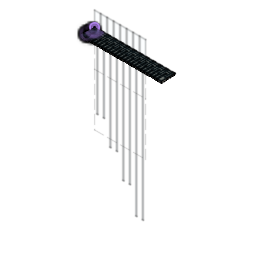
model (Autodesk Fusion 360 design; units mm, degrees)
Autodesk Fusion 360 part; units mm, degrees
sketch "kre" plane through (0, 0, 0) normal (0, 1, 0) x (1, 0, 0) in component "sketches"
  line L0 (20.5, 670) -> (29.5, 670)
  line L1 (29.5, 670) -> (29.5, 0)
  line L2 (29.5, 0) -> (20.5, 0)
  line L3 (20.5, 0) -> (20.5, 670)
  line L4 (0, 0) -> (50, 0)
  line L5 (50, 0) -> (50, -135)
  line L6 (50, -135) -> (0, -135)
  line L7 (0, -135) -> (0, 0)
  line L8 (109, 0) -> (109, -135)
  line L9 (109, -135) -> (59, -135)
  line L10 (59, -135) -> (59, 0)
  line L11 (59, 0) -> (109, 0)
  line L12 (88.5, 670) -> (88.5, 0)
  line L13 (88.5, 0) -> (79.5, 0)
  line L14 (79.5, 670) -> (88.5, 670)
  line L15 (79.5, 0) -> (79.5, 670)
  line L16 (168, 0) -> (168, -135)
  line L17 (168, -135) -> (118, -135)
  line L18 (118, -135) -> (118, 0)
  line L19 (118, 0) -> (168, 0)
  line L20 (147.5, 872) -> (147.5, 0)
  line L21 (147.5, 0) -> (138.5, 0)
  line L22 (138.5, 872) -> (147.5, 872)
  line L23 (138.5, 0) -> (138.5, 872)
  line L24 (227, 0) -> (227, -135)
  line L25 (227, -135) -> (177, -135)
  line L26 (177, -135) -> (177, 0)
  line L27 (177, 0) -> (227, 0)
  line L28 (206.5, 872) -> (206.5, 0)
  line L29 (206.5, 0) -> (197.5, 0)
  line L30 (197.5, 872) -> (206.5, 872)
  line L31 (197.5, 0) -> (197.5, 872)
  line L32 (286, 0) -> (286, -135)
  line L33 (286, -135) -> (236, -135)
  line L34 (236, -135) -> (236, 0)
  line L35 (236, 0) -> (286, 0)
  line L36 (265.5, 1074) -> (265.5, 0)
  line L37 (265.5, 0) -> (256.5, 0)
  line L38 (256.5, 1074) -> (265.5, 1074)
  line L39 (256.5, 0) -> (256.5, 1074)
  line L40 (345, 0) -> (345, -135)
  line L41 (345, -135) -> (295, -135)
  line L42 (295, -135) -> (295, 0)
  line L43 (295, 0) -> (345, 0)
  line L44 (324.5, 1074) -> (324.5, 0)
  line L45 (324.5, 0) -> (315.5, 0)
  line L46 (315.5, 1074) -> (324.5, 1074)
  line L47 (315.5, 0) -> (315.5, 1074)
  line L48 (404, 0) -> (404, -135)
  line L49 (404, -135) -> (354, -135)
  line L50 (354, -135) -> (354, 0)
  line L51 (354, 0) -> (404, 0)
  line L52 (383.5, 1295) -> (383.5, 0)
  line L53 (383.5, 0) -> (374.5, 0)
  line L54 (374.5, 1295) -> (383.5, 1295)
  line L55 (374.5, 0) -> (374.5, 1295)
  line L56 (463, 0) -> (463, -135)
  line L57 (463, -135) -> (413, -135)
  line L58 (413, -135) -> (413, 0)
  line L59 (413, 0) -> (463, 0)
  line L60 (442.5, 1295) -> (442.5, 0)
  line L61 (442.5, 0) -> (433.5, 0)
  line L62 (433.5, 1295) -> (442.5, 1295)
  line L63 (433.5, 0) -> (433.5, 1295)
  line L64 (50, 0) -> (59, 0) construction
  line L65 (109, 0) -> (118, 0) construction
  line L66 (168, 0) -> (177, 0) construction
  line L67 (227, 0) -> (236, 0) construction
  line L68 (286, 0) -> (295, 0) construction
  line L69 (345, 0) -> (354, 0) construction
  line L70 (404, 0) -> (413, 0) construction
  line L71 (0, 0) -> (463, 0) construction
  line L72 (463, 0) -> (463, 130) construction
  line L73 (463, 130) -> (0, 130) construction
  line L74 (0, 130) -> (0, 0) construction
  line L75 (0, 130) -> (0, 330) construction
  line L76 (0, 330) -> (463, 330) construction
  line L77 (463, 330) -> (463, 130) construction
  line L78 (0, 330) -> (0, 807) construction
  line L79 (0, 807) -> (463, 807) construction
  line L80 (463, 807) -> (463, 330) construction
  dimension "d1" = 135
  dimension "d2" = 50
  dimension "d3" = 805
  dimension "d4" = 9
  dimension "d5" = 135
  dimension "d6" = 50
  dimension "d7" = 805
  dimension "d8" = 9
  dimension "d9" = 135
  dimension "d10" = 50
  dimension "d11" = 1007
  dimension "d12" = 9
  dimension "d13" = 135
  dimension "d14" = 50
  dimension "d15" = 1007
  dimension "d16" = 9
  dimension "d17" = 135
  dimension "d18" = 50
  dimension "d19" = 1209
  dimension "d20" = 9
  dimension "d21" = 135
  dimension "d22" = 50
  dimension "d23" = 1209
  dimension "d24" = 9
  dimension "d25" = 135
  dimension "d26" = 50
  dimension "d27" = 1430
  dimension "d28" = 9
  dimension "d29" = 135
  dimension "d30" = 50
  dimension "d31" = 1430
  dimension "d32" = 9
  dimension "d34" = 50
  dimension "d35" = 130
  dimension "d56" = 200
  dimension "d57" = 677
  constraint horizontal L0
  constraint vertical L1
  constraint horizontal L2
  constraint vertical L3
  constraint horizontal L4
  constraint vertical L5
  constraint horizontal L6
  constraint vertical L7
  constraint midpoint L2 L4
  constraint horizontal L14
  constraint vertical L12
  constraint horizontal L13
  constraint vertical L15
  constraint horizontal L11
  constraint vertical L8
  constraint horizontal L9
  constraint vertical L10
  constraint midpoint L11 L13
  constraint horizontal L22
  constraint vertical L20
  constraint horizontal L21
  constraint vertical L23
  constraint horizontal L19
  constraint vertical L16
  constraint horizontal L17
  constraint vertical L18
  constraint midpoint L19 L21
  constraint horizontal L30
  constraint vertical L28
  constraint horizontal L29
  constraint vertical L31
  constraint horizontal L27
  constraint vertical L24
  constraint horizontal L25
  constraint vertical L26
  constraint midpoint L27 L29
  constraint horizontal L38
  constraint vertical L36
  constraint horizontal L37
  constraint vertical L39
  constraint horizontal L35
  constraint vertical L32
  constraint horizontal L33
  constraint vertical L34
  constraint midpoint L35 L37
  constraint horizontal L46
  constraint vertical L44
  constraint horizontal L45
  constraint vertical L47
  constraint horizontal L43
  constraint vertical L40
  constraint horizontal L41
  constraint vertical L42
  constraint midpoint L43 L45
  constraint horizontal L54
  constraint vertical L52
  constraint horizontal L53
  constraint vertical L55
  constraint horizontal L51
  constraint vertical L48
  constraint horizontal L49
  constraint vertical L50
  constraint midpoint L51 L53
  constraint horizontal L62
  constraint vertical L60
  constraint horizontal L61
  constraint vertical L63
  constraint horizontal L59
  constraint vertical L56
  constraint horizontal L57
  constraint vertical L58
  constraint midpoint L59 L61
  constraint collinear L6 L9
  constraint collinear L9 L17
  constraint collinear L17 L25
  constraint collinear L25 L33
  constraint collinear L33 L41
  constraint collinear L41 L49
  constraint collinear L49 L57
  constraint coincident L4.start L7.end
  constraint equal L64 L65
  constraint equal L65 L66
  constraint equal L66 L67
  constraint equal L67 L68
  constraint equal L68 L69
  constraint equal L69 L70
  constraint horizontal L71
  constraint vertical L72
  constraint horizontal L73
  constraint vertical L74
  constraint collinear L56 L72
  constraint vertical L77
  constraint vertical L75
  constraint horizontal L76
  constraint horizontal L79
  constraint vertical L80
  constraint vertical L78
  measures "d1" distance of L4.end L5.end
  measures "d2" distance of L5.end L6.end
  measures "d3" distance of L0 L6
  measures "d4" distance of L1 L3
  measures "d5" distance of L8.start L8.end
  measures "d6" distance of L9.end L8.end
  measures "d7" distance of L9 L14
  measures "d8" distance of L12 L15
  measures "d9" distance of L16.start L16.end
  measures "d10" distance of L17.end L16.end
  measures "d11" distance of L17 L22
  measures "d12" distance of L20 L23
  measures "d13" distance of L24.start L24.end
  measures "d14" distance of L25.end L24.end
  measures "d15" distance of L25 L30
  measures "d16" distance of L28 L31
  measures "d17" distance of L32.start L32.end
  measures "d18" distance of L33.end L32.end
  measures "d19" distance of L33 L38
  measures "d20" distance of L36 L39
  measures "d21" distance of L40.start L40.end
  measures "d22" distance of L41.end L40.end
  measures "d23" distance of L41 L46
  measures "d24" distance of L44 L47
  measures "d25" distance of L48.start L48.end
  measures "d26" distance of L49.end L48.end
  measures "d27" distance of L49 L54
  measures "d28" distance of L52 L55
  measures "d29" distance of L56.start L56.end
  measures "d30" distance of L57.end L56.end
  measures "d31" distance of L57 L62
  measures "d32" distance of L60 L63
  measures "d34" distance of L1 L15
  measures "d35" distance of L56.start L72.end
  measures "d56" distance of L73 L76
  measures "d57" distance of L73 L79
sketch "profile" plane through (0, 0, 0) normal (0, 0, 1) x (1, 0, 0) in component "rack"
  line L0 (0, 0) -> (726, 0)
  line L1 (726, 0) -> (726, -120)
  line L2 (726, -120) -> (0, -120)
  line L3 (0, -120) -> (0, 0)
  line L4 (33.5, -120) -> (43.5, -120)
  line L5 (43.5, -120) -> (43.5, -40)
  line L6 (43.5, -40) -> (33.5, -40)
  line L7 (33.5, -40) -> (33.5, -120)
  line L8 (92.5, -40) -> (92.5, -120)
  line L9 (92.5, -120) -> (102.5, -120)
  line L10 (102.5, -40) -> (92.5, -40)
  line L11 (102.5, -120) -> (102.5, -40)
  line L12 (151.5, -40) -> (151.5, -120)
  line L13 (151.5, -120) -> (161.5, -120)
  line L14 (161.5, -40) -> (151.5, -40)
  line L15 (161.5, -120) -> (161.5, -40)
  line L16 (210.5, -40) -> (210.5, -120)
  line L17 (210.5, -120) -> (220.5, -120)
  line L18 (220.5, -40) -> (210.5, -40)
  line L19 (220.5, -120) -> (220.5, -40)
  line L20 (269.5, -40) -> (269.5, -120)
  line L21 (269.5, -120) -> (279.5, -120)
  line L22 (279.5, -40) -> (269.5, -40)
  line L23 (279.5, -120) -> (279.5, -40)
  line L24 (328.5, -40) -> (328.5, -120)
  line L25 (328.5, -120) -> (338.5, -120)
  line L26 (338.5, -40) -> (328.5, -40)
  line L27 (338.5, -120) -> (338.5, -40)
  line L28 (387.5, -40) -> (387.5, -120)
  line L29 (387.5, -120) -> (397.5, -120)
  line L30 (397.5, -40) -> (387.5, -40)
  line L31 (397.5, -120) -> (397.5, -40)
  line L32 (446.5, -40) -> (446.5, -120)
  line L33 (446.5, -120) -> (456.5, -120)
  line L34 (456.5, -40) -> (446.5, -40)
  line L35 (456.5, -120) -> (456.5, -40)
  line L36 (505.5, -40) -> (505.5, -120)
  line L37 (505.5, -120) -> (515.5, -120)
  line L38 (515.5, -40) -> (505.5, -40)
  line L39 (515.5, -120) -> (515.5, -40)
  line L40 (564.5, -40) -> (564.5, -120)
  line L41 (564.5, -120) -> (574.5, -120)
  line L42 (574.5, -40) -> (564.5, -40)
  line L43 (574.5, -120) -> (574.5, -40)
  line L44 (623.5, -40) -> (623.5, -120)
  line L45 (623.5, -120) -> (633.5, -120)
  line L46 (633.5, -40) -> (623.5, -40)
  line L47 (633.5, -120) -> (633.5, -40)
  line L48 (682.5, -40) -> (682.5, -120)
  line L49 (682.5, -120) -> (692.5, -120)
  line L50 (692.5, -40) -> (682.5, -40)
  line L51 (692.5, -120) -> (692.5, -40)
  line L52 (63.75, -120) -> (72.25, -120)
  line L53 (72.25, -120) -> (72.25, -75)
  line L54 (72.25, -75) -> (63.75, -75)
  line L55 (63.75, -75) -> (63.75, -120)
  line L56 (63.75, -97.5) -> (43.5, -97.5) construction
  line L57 (72.25, -97.5) -> (92.5, -97.5) construction
  line L58 (122.75, -75) -> (122.75, -120)
  line L59 (122.75, -120) -> (131.25, -120)
  line L60 (131.25, -75) -> (122.75, -75)
  line L61 (131.25, -120) -> (131.25, -75)
  line L62 (181.75, -75) -> (181.75, -120)
  line L63 (181.75, -120) -> (190.25, -120)
  line L64 (190.25, -75) -> (181.75, -75)
  line L65 (190.25, -120) -> (190.25, -75)
  line L66 (240.75, -75) -> (240.75, -120)
  line L67 (240.75, -120) -> (249.25, -120)
  line L68 (249.25, -75) -> (240.75, -75)
  line L69 (249.25, -120) -> (249.25, -75)
  line L70 (299.75, -75) -> (299.75, -120)
  line L71 (299.75, -120) -> (308.25, -120)
  line L72 (308.25, -75) -> (299.75, -75)
  line L73 (308.25, -120) -> (308.25, -75)
  line L74 (358.75, -75) -> (358.75, -120)
  line L75 (358.75, -120) -> (367.25, -120)
  line L76 (367.25, -75) -> (358.75, -75)
  line L77 (367.25, -120) -> (367.25, -75)
  line L78 (417.75, -75) -> (417.75, -120)
  line L79 (417.75, -120) -> (426.25, -120)
  line L80 (426.25, -75) -> (417.75, -75)
  line L81 (426.25, -120) -> (426.25, -75)
  line L82 (476.75, -75) -> (476.75, -120)
  line L83 (476.75, -120) -> (485.25, -120)
  line L84 (485.25, -75) -> (476.75, -75)
  line L85 (485.25, -120) -> (485.25, -75)
  line L86 (535.75, -75) -> (535.75, -120)
  line L87 (535.75, -120) -> (544.25, -120)
  line L88 (544.25, -75) -> (535.75, -75)
  line L89 (544.25, -120) -> (544.25, -75)
  line L90 (594.75, -75) -> (594.75, -120)
  line L91 (594.75, -120) -> (603.25, -120)
  line L92 (603.25, -75) -> (594.75, -75)
  line L93 (603.25, -120) -> (603.25, -75)
  line L94 (653.75, -75) -> (653.75, -120)
  line L95 (653.75, -120) -> (662.25, -120)
  line L96 (662.25, -75) -> (653.75, -75)
  line L97 (662.25, -120) -> (662.25, -75)
  line L98 (59, 0) -> (77, 0)
  line L99 (77, 0) -> (77, -70)
  line L100 (77, -70) -> (59, -70)
  line L101 (59, -70) -> (59, 0)
  line L102 (43.5, -40) -> (59, -40) construction
  line L103 (92.5, -40) -> (77, -40) construction
  line L104 (136, 0) -> (136, -70)
  line L105 (136, -70) -> (118, -70)
  line L106 (118, 0) -> (136, 0)
  line L107 (118, -70) -> (118, 0)
  line L108 (195, 0) -> (195, -70)
  line L109 (195, -70) -> (177, -70)
  line L110 (177, 0) -> (195, 0)
  line L111 (177, -70) -> (177, 0)
  line L112 (254, 0) -> (254, -70)
  line L113 (254, -70) -> (236, -70)
  line L114 (236, 0) -> (254, 0)
  line L115 (236, -70) -> (236, 0)
  line L116 (313, 0) -> (313, -70)
  line L117 (313, -70) -> (295, -70)
  line L118 (295, 0) -> (313, 0)
  line L119 (295, -70) -> (295, 0)
  line L120 (372, 0) -> (372, -70)
  line L121 (372, -70) -> (354, -70)
  line L122 (354, 0) -> (372, 0)
  line L123 (354, -70) -> (354, 0)
  line L124 (431, 0) -> (431, -70)
  line L125 (431, -70) -> (413, -70)
  line L126 (413, 0) -> (431, 0)
  line L127 (413, -70) -> (413, 0)
  line L128 (490, 0) -> (490, -70)
  line L129 (490, -70) -> (472, -70)
  line L130 (472, 0) -> (490, 0)
  line L131 (472, -70) -> (472, 0)
  line L132 (549, 0) -> (549, -70)
  line L133 (549, -70) -> (531, -70)
  line L134 (531, 0) -> (549, 0)
  line L135 (531, -70) -> (531, 0)
  line L136 (608, 0) -> (608, -70)
  line L137 (608, -70) -> (590, -70)
  line L138 (590, 0) -> (608, 0)
  line L139 (590, -70) -> (590, 0)
  line L140 (667, 0) -> (667, -70)
  line L141 (667, -70) -> (649, -70)
  line L142 (649, 0) -> (667, 0)
  line L143 (649, -70) -> (649, 0)
  line L144 (0, 0) -> (18, 0)
  line L145 (18, 0) -> (18, -70)
  line L146 (18, -70) -> (0, -70)
  line L147 (0, -70) -> (0, 0)
  line L148 (726, 0) -> (708, 0)
  line L149 (708, 0) -> (708, -70)
  line L150 (708, -70) -> (726, -70)
  line L151 (726, -70) -> (726, 0)
  line L152 (33.5, -40) -> (18, -40) construction
  line L153 (692.5, -40) -> (708, -40) construction
  line L154 (0, -18) -> (726, -18)
  line L155 (33.5, -18) -> (33.5, 0) construction
  dimension "d38" = 120
  dimension "d41" = 10
  dimension "d42" = 40
  dimension "d45" = 59
  dimension "d46" = 0
  dimension "d47" = 8.5
  dimension "d48" = 75
  dimension "d51" = 59
  dimension "d52" = 0
  dimension "d58" = 18
  dimension "d59" = 5
  dimension "d60" = 70
  dimension "d63" = 59
  dimension "d64" = 0
  constraint horizontal L0
  constraint vertical L1
  constraint horizontal L2
  constraint vertical L3
  constraint coincident L0.start L3.end
  constraint horizontal L4
  constraint vertical L5
  constraint horizontal L6
  constraint vertical L7
  constraint coincident L2 L4.start
  constraint horizontal L52
  constraint vertical L53
  constraint horizontal L54
  constraint vertical L55
  constraint coincident L2 L52.start
  constraint midpoint L55 L56.start
  constraint coincident L5 L56.end
  constraint perpendicular L5 L56
  constraint midpoint L53 L57.start
  constraint coincident L8 L57.end
  constraint perpendicular L8 L57
  constraint equal L56 L57
  constraint horizontal L98
  constraint vertical L99
  constraint horizontal L100
  constraint vertical L101
  constraint coincident L0 L98.start
  constraint coincident L101 L102.end
  constraint coincident L99 L103.end
  constraint equal L102 L103
  constraint horizontal L102
  constraint horizontal L103
  constraint horizontal L144
  constraint vertical L145
  constraint horizontal L146
  constraint vertical L147
  constraint equal L100 L146
  constraint equal L101 L145
  constraint horizontal L148
  constraint vertical L149
  constraint horizontal L150
  constraint vertical L151
  constraint equal L101 L149
  constraint equal L100 L150
  constraint coincident L145 L152.end
  constraint perpendicular L145 L152
  constraint equal L102 L152
  constraint coincident L149 L153.end
  constraint perpendicular L149 L153
  constraint equal L152 L153
  constraint coincident L147 L154.start
  constraint coincident L151 L154.end
  constraint horizontal L154
  constraint coincident L154 L155.start
  constraint coincident L0 L155.end
  constraint perpendicular L0 L155
  constraint equal L100 L155
  constraint collinear L7 L155
  measures "d38" distance of L0 L2
  measures "d41" distance of L5.end L6.end
  measures "d42" distance of L0 L6
  measures "d47" distance of L53.end L54.end
  measures "d48" distance of L0 L54
  measures "d58" distance of L99 L101
  measures "d59" distance of L54 L100
  measures "d60" distance of L98.start L100.end
extrude "Extrude1" add sketch "profile" against normal blind 18 contours L0 L3 L144 L145 L147 L154 | L0 L101 L145 L154 | L3 L145 L146 L147 L154 | L0 L98 L99 L101 L154 | L1 L2 L3 L5 L6 L7 L8 L10 L11 L12 L14 L15 L16 L18 L19 L20 L22 L23 L24 L26 L27 L28 L30 L31 L32 L34 L35 L36 L38 L39 L40 L42 L43 L44 L46 L47 L48 L50 L51 L53 L54 L55 L58 L60 L61 L62 L64 L65 L66 L68 L69 L70 L72 L73 L74 L76 L77 L78 L80 L81 L82 L84 L85 L86 L88 L89 L90 L92 L93 L94 L96 L97 L99 L100 L101 L104 L105 L107 L108 L109 L111 L112 L113 L115 L116 L117 L119 L120 L121 L123 L124 L125 L127 L128 L129 L131 L132 L133 L135 L136 L137 L139 L140 L141 L143 L145 L146 L149 L150 L154 | L0 L99 L107 L154 | L99 L100 L101 L154 | L0 L104 L106 L107 L154 | L0 L104 L111 L154 | L104 L105 L107 L154 | L0 L108 L110 L111 L154 | L0 L108 L115 L154 | L108 L109 L111 L154 | L0 L112 L114 L115 L154 | L0 L112 L119 L154 | L112 L113 L115 L154 | L0 L116 L118 L119 L154 | L0 L116 L123 L154 | L116 L117 L119 L154 | L0 L120 L122 L123 L154 | L0 L120 L127 L154 | L120 L121 L123 L154 | L0 L124 L126 L127 L154 | L0 L124 L131 L154 | L124 L125 L127 L154 | L0 L128 L130 L131 L154 | L0 L128 L135 L154 | L128 L129 L131 L154 | L0 L132 L134 L135 L154 | L0 L132 L139 L154 | L132 L133 L135 L154 | L0 L136 L138 L139 L154 | L0 L136 L143 L154 | L136 L137 L139 L154 | L0 L140 L142 L143 L154 | L0 L140 L149 L154 | L140 L141 L143 L154 | L0 L1 L148 L149 L151 L154 | L1 L149 L150 L151 L154 makes body 1 in component "rack"
extrude "Extrude2" cut sketch "profile" along normal blind 4 from surface at -18 contours L0 L3 L144 L145 L147 L154 | L0 L101 L145 L154 | L3 L145 L146 L147 L154 | L0 L98 L99 L101 L154 | L0 L99 L107 L154 | L99 L100 L101 L154 | L0 L104 L106 L107 L154 | L0 L104 L111 L154 | L104 L105 L107 L154 | L0 L108 L110 L111 L154 | L0 L108 L115 L154 | L108 L109 L111 L154 | L0 L112 L114 L115 L154 | L0 L112 L119 L154 | L112 L113 L115 L154 | L0 L116 L118 L119 L154 | L0 L116 L123 L154 | L116 L117 L119 L154 | L0 L120 L122 L123 L154 | L0 L120 L127 L154 | L120 L121 L123 L154 | L0 L124 L126 L127 L154 | L0 L124 L131 L154 | L124 L125 L127 L154 | L0 L128 L130 L131 L154 | L0 L128 L135 L154 | L128 L129 L131 L154 | L0 L132 L134 L135 L154 | L0 L132 L139 L154 | L132 L133 L135 L154 | L0 L136 L138 L139 L154 | L0 L136 L143 L154 | L136 L137 L139 L154 | L0 L140 L142 L143 L154 | L0 L140 L149 L154 | L140 L141 L143 L154 | L0 L1 L148 L149 L151 L154 | L1 L149 L150 L151 L154 bodies 1 in component "rack"
sketch "support" plane through (0, 0, 0) normal (-1, 0, 0) x (0, -1, 0) in component "rack"
  line L0 (70, -14) -> (70, -18)
  line L1 (70, -18) -> (120, -18)
  line L2 (120, -18) -> (120, 0)
  line L3 (120, 0) -> (0, 0)
  line L4 (0, 0) -> (0, -14)
  line L5 (0, -14) -> (70, -14)
  line L6 (18, -18) -> (70, -18)
  line L7 (70, -18) -> (70, -14)
  line L8 (70, -14) -> (18, -14)
  line L9 (18, -14) -> (18, -18)
  line L10 (14, -70) -> (18, -70)
  line L11 (18, -70) -> (70, -18)
  line L12 (14, -70) -> (14, -14)
  line L13 (18, -18) -> (18, -70) construction
  arc A0 (18, -70) -> (25.0711, -67.0711) centre (18, -60) ccw
  arc A1 (67.0711, -25.0711) -> (70, -18) centre (60, -18) ccw
  line L14 (25.0711, -67.0711) -> (67.0711, -25.0711)
  dimension "d73" = 10
  constraint coincident L0.end L1.start
  constraint equal L0 L10
  constraint coincident L5 L12.end
  constraint coincident L6.start L9.end
  constraint parallel L12 L13
  constraint vertical L12
  constraint equal L6 L13
  constraint horizontal L10
  constraint tangent L10 A0
  constraint tangent L7 A1
  constraint tangent A0 L14
  constraint tangent A1 L14
  constraint equal A0 A1
  measures "d73" radius of A0
extrude "Extrude3" add sketch "support" against normal blind 18 separate body contours L0 L5 L6 L7 L8 L9 | L5 L6 L9 L10 L11 L12 | L11 A0 A1 L14 makes body 2 in component "rack"
component "sketches" placed x (1, 0, 0) y (0, 1, 0) z (0, 0, 1) at (0, 0, 0)
component "rack" placed x (1, 0, 0) y (0, 1, 0) z (0, 0, 1) at (0, 0, 0)
equation "d45 = kreSpacing"
equation "d51 = kreSpacing"
equation "kreSpacing = 59 mm"
equation "d58 = plyT"
equation "d63 = kreSpacing"
equation "dado = 4 mm"
equation "d67 = dado"
equation "plyT = 18 mm"
